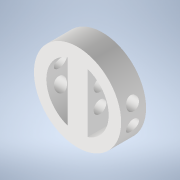
# Autodesk Inventor part: FahnenhalterTeiloben
Saved by Autodesk Inventor 2020.3 (Build 243373010, 373A)
## iProperties
Created: 2020-10-20
Part Number: FahnenhalterTeiloben
Material: Generisch
Document SubType Name: Modeling
Designer: Stefan
Density: 1 g/cm^3
Appearance: Vorgabe
Author: Stefan
Autodesk Inventor part; units mm, degrees
ref_plane "YZ Plane" through (0, 0, 0) normal (1, 0, 0) x (0, 1, 0)
ref_plane "XZ Plane" through (0, 0, 0) normal (0, 1, 0) x (-1, 0, 0)
ref_plane "XY Plane" through (0, 0, 0) normal (0, 0, 1) x (1, 0, 0)
sketch "Skizze1" plane through (0, 0, 0) normal (0, 0, 1) x (1, 0, 0)
  circle A0 centre (0, 0) radius 17.5
  circle A1 centre (0, 0) radius 12.5 construction
  line L0 (-4, 11.8427) -> (4, 11.8427) construction
  line L1 (4, 11.8427) -> (4, -11.8427)
  line L2 (4, -11.8427) -> (-4, -11.8427) construction
  line L3 (-4, -11.8427) -> (-4, 11.8427)
  arc A2 (-4, 11.8427) -> (-4, -11.8427) centre (0, 0) ccw
  arc A3 (4, -11.8427) -> (4, 11.8427) centre (0, 0) ccw
  dimension "d0" = 35
  dimension "d1" = 25
  dimension "d2" = 8
  dimension "d3" = 4
  dimension "d4" = 25
  dimension "d5" = 0
  constraints: 8 end point, 7 point on circle, 4 centre point, 4 coincident, 2 parallel, 1 horizontal, 1 perpendicular
  measures "d0" diameter of A0
  measures "d1" diameter of A1
  measures "d2" distance of L1.end L2.end
  measures "d3" distance from line of L1 point (0, 0)
  measures "d4" distance of L1.end L0.start
  measures "d5" distance of L2.end A2.end
extrude "Extrusion1" add sketch "Skizze1" along normal blind 10
sketch "Skizze2" plane through (4, -11.8427, 0) normal (1, 0, 0) x (0, 0, -1)
  circle A0 centre (-5, 15.6854) radius 2.525
  circle A1 centre (-5, 8) radius 2.525
  line L0 (0, 0) -> (-10, 0) projected
  line L1 (0, 23.6854) -> (-10, 23.6854) projected
  line L2 (-10, 0) -> (-10, 23.6854) projected
  point P0 (0, 11.8427)
  dimension "d8" = 5.05
  dimension "d9" = 5.05
  dimension "d10" = 8
  dimension "d11" = 8
  dimension "d12" = 5
  dimension "d13" = 5
  constraints: 2 centre point
  measures "d8" diameter of A0
  measures "d9" diameter of A1
  measures "d10" distance from line of L0 A1.centre
  measures "d11" distance from line of A0.centre L1
  measures "d12" distance from line of L2 A0.centre
  measures "d13" distance from line of L2 A1.centre
extrude "Extrusion2" cut sketch "Skizze2" along normal mid plane 500
